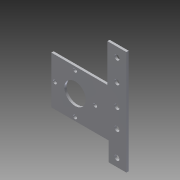
# Autodesk Inventor part: p80 mount plate
Saved by Autodesk Inventor 2013 (Build 170138000, 138)
## iProperties
Created: 2013-01-31
Part Number: p80 mount plate
Material: Aluminum 6061
Document SubType Name: Sheet Metal
Designer: Arpan
Density: 2.71 g/cm^3
Sheet Metal Rule: Default
Mass: 44.9973 g
Surface Area: 125.822 cm^2
Volume: 16.6042 cm^3
Author: Arpan
Autodesk Inventor part; units mm, degrees
ref_plane "YZ Plane" through (0, 0, 0) normal (1, 0, 0) x (0, 1, 0)
ref_plane "XZ Plane" through (0, 0, 0) normal (0, 1, 0) x (-1, 0, 0)
ref_plane "XY Plane" through (0, 0, 0) normal (0, 0, 1) x (1, 0, 0)
sketch "Sketch1" plane through (0, 0, 0) normal (0, 0, 1) x (1, 0, 0)
  line L0 (0, 0) -> (-63.5, 0)
  line L1 (-63.5, 0) -> (-63.5, 63.5)
  line L2 (-63.5, 63.5) -> (0, 63.5)
  circle A0 centre (-58.7502, 31.75) radius 2.54
  circle A1 centre (-31.75, 58.7502) radius 2.54
  circle A2 centre (-4.7498, 31.75) radius 2.54
  circle A3 centre (-31.75, 4.7498) radius 2.54
  line L3 (36.9316, 63.5) -> (36.9316, 0)
  line L4 (13.1168, 0) -> (0, 0)
  circle A4 centre (-31.75, 31.75) radius 14.2875
  line L5 (24.2316, 63.5) -> (24.2316, 44.45)
  line L6 (24.2316, 44.45) -> (24.2316, 19.05)
  circle A5 centre (24.2316, 44.45) radius 3.3782
  circle A6 centre (24.2316, 19.05) radius 3.3782
  line L7 (20.8534, 44.45) -> (20.8534, 19.05)
  line L8 (27.6098, 19.05) -> (27.6098, 44.45)
  line L9 (11.5316, 63.5) -> (11.5316, 114.3)
  line L10 (13.1168, 0) -> (13.1168, -25.4)
  line L11 (13.1168, -25.4) -> (36.9316, -25.4)
  line L12 (36.9316, -25.4) -> (36.9316, 0)
  line L13 (11.5316, 114.3) -> (36.9316, 114.3)
  line L14 (36.9316, 114.3) -> (36.9316, 63.5)
  line L15 (0, 63.5) -> (11.5316, 63.5)
  dimension "d0" = 63.5
  dimension "d1" = 63.5
  dimension "d6" = 5.08
  dimension "d7" = 5.08
  dimension "d8" = 5.08
  dimension "d9" = 5.08
  dimension "d11" = 36.9316
  dimension "d12" = 28.575
  dimension "d13" = 12.7
  dimension "d15" = 25.4
  dimension "d16" = 6.7564
  dimension "d17" = 6.7564
  dimension "d23" = 50.8
  dimension "d24" = 25.4
  measures "d0" distance of L0.start L0.end
  measures "d1" distance of L0.end L1.end
  measures "d6" diameter of A0
  measures "d7" diameter of A1
  measures "d8" diameter of A2
  measures "d9" diameter of A3
  measures "d11" distance of L2.end L3.start
  measures "d12" diameter of A4
  measures "d13" distance of L5.start L3.start
  measures "d15" distance of L5.end L6.end
  measures "d16" diameter of A5
  measures "d17" diameter of A6
  measures "d23" distance of L9.start L9.end
  measures "d24" distance of L4.start L10.end
extrude "Plate2" add sketch "Sketch1" along normal blind 3.048 contours L0 L1 L2 L15 L9 L13 L14 L3 L12 L11 L10 L4 | L8 A6 L6 A5 | A5 L6 A6 L7
sketch "Sketch4" plane through (0, 0, 3.048) normal (0, 0, 1) x (1, 0, 0)
  circle A0 centre (24.2316, 19.05) radius 3.3782 projected
  circle A1 centre (24.2316, 44.45) radius 3.3782 projected
  line L0 (-63.5, 63.5) -> (11.5316, 63.5) projected
  line L1 (24.2316, 44.45) -> (24.2316, 101.6)
  circle A2 centre (24.2316, 101.6) radius 3.3782
  circle A3 centre (24.2316, 73.025) radius 3.3782
  line L2 (24.2316, 19.05) -> (24.2316, -14.605)
  circle A4 centre (24.2316, -14.605) radius 3.3782
  point P0 (0, 0)
  point P1 (20.8534, 44.45)
  point P2 (20.8534, 19.05)
  point P3 (27.6098, 19.05)
  point P4 (27.6098, 44.45)
  dimension "d25" = 57.15
  dimension "d26" = 6.7564
  dimension "d27" = 6.7564
  dimension "d28" = 33.655
  dimension "d29" = 6.7564
  constraints: 4 end point, 4 point on circle, 3 centre point, 2 coincident, 1 collinear, 1 midpoint, 1 perpendicular
  measures "d25" distance of L1.start L1.end
  measures "d26" diameter of A2
  measures "d27" diameter of A3
  measures "d28" distance of L2.start L2.end
  measures "d29" diameter of A4
extrude "Cut1" cut sketch "Sketch4" against normal blind 3.048
fillet "Corner Round1" radius 19.05 2 edges at (11.5316, 63.5, 1.524) (13.1168, 0, 1.524)
fillet "Corner Round2" radius 6.35 6 edges at (-63.5, 63.5, 1.524) (-63.5, 0, 1.524) (13.1168, -25.4, 1.524) (36.9316, -25.4, 1.524) (36.9316, 114.3, 1.524) (11.5316, 114.3, 1.524)
equation "\"d19\" = Thickness"
equation "\"BendRadius\" = Thickness"
equation "\"BendReliefWidth\" = Thickness"
equation "\"BendReliefDepth\" = 0.5 * Thickness"
equation "\"CornerReliefSize\" = 4 * Thickness"
equation "\"MinimumRemnant\" = 2 * Thickness"
equation "\"TransitionRadius\" = BendRadius"
equation "\"JacobiRadiusSize\" = BendRadius"
equation "\"GapSize\" = Thickness"
equation "\"d10\" = BendRadius"
equation "\"d18\" = BendRadius"
equation "\"Thickness\" = 3.048"
body "Solid2"
